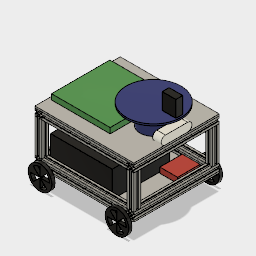
TEST AREA Body (v1~recovered) (Autodesk Fusion 360 design; units mm, degrees)
Autodesk Fusion 360 part; units mm, degrees
sketch "Sketch1" plane through (0, 0, 0) normal (0, 1, 0) x (1, 0, 0)
  line L0 (0, 0) -> (20, 0)
  line L1 (20, 0) -> (20, -20)
  line L2 (20, -20) -> (0, -20)
  line L3 (0, -20) -> (0, 0)
  line L4 (14, -14) -> (6, -14)
  line L5 (6, -14) -> (6, -6)
  line L6 (6, -6) -> (14, -6)
  line L7 (14, -6) -> (14, -14)
  line L8 (14, -14) -> (6, -6) construction
  line L9 (6, -14) -> (14, -6) construction
  circle A0 centre (10, -10) radius 2.1
  line L10 (10, 0) -> (13, 0)
  line L11 (10, 0) -> (7, 0)
  line L12 (7, 0) -> (7, -2)
  line L13 (13, 0) -> (13, -2)
  line L14 (13, -2) -> (10, -2)
  line L15 (13, -2) -> (16, -2)
  line L16 (7, -2) -> (4, -2)
  line L17 (2, -7) -> (2, -4)
  line L18 (0, -7) -> (2, -7)
  line L19 (0, -13) -> (2, -13)
  line L20 (2, -13) -> (2, -16)
  line L21 (7, -18) -> (4, -18)
  line L22 (7, -20) -> (7, -18)
  line L23 (13, -20) -> (13, -18)
  line L24 (13, -18) -> (16, -18)
  line L25 (18, -13) -> (18, -16)
  line L26 (20, -13) -> (18, -13)
  line L27 (20, -7) -> (18, -7)
  line L28 (18, -7) -> (18, -4)
  line L29 (18, -4) -> (4, -18)
  line L30 (2, -16) -> (16, -2)
  line L31 (18, -16) -> (4, -2)
  line L32 (2, -4) -> (16, -18)
  point P0 (10, -10)
  dimension "d1" = 20
  dimension "d2" = 20
  dimension "d3" = 8
  dimension "d4" = 8
  dimension "d5" = 4.2
  dimension "d6" = 3
  dimension "d7" = 3
  dimension "d8" = 2
  dimension "d9" = 2
  dimension "d11" = 360
  measures "d1" distance of L0.start L0.end
  measures "d2" distance of L0.start L2.end
  measures "d3" distance of L4.end L5.end
  measures "d4" distance of L5.end L6.end
  measures "d5" diameter of A0
  measures "d6" distance of L10.start L10.end
  measures "d7" distance of L10.start L11.end
  measures "d8" distance of L11.end L12.end
  measures "d9" distance of L10.end L13.end
extrude "Extrude1" add sketch "Sketch1" along normal blind 19 contours L0 L3 L5 L6 L12 L16 L17 L18 L31 L32 | L2 L3 L4 L5 L19 L20 L21 L22 L29 L30 | L0 L1 L6 L7 L13 L15 L27 L28 L29 L30 | L5 L6 A0 L31 L32 | L6 A0 L30 L31 | L5 A0 L30 L32 | L6 L7 A0 L29 L30 | L1 L2 L4 L7 L23 L24 L25 L26 L31 L32 | L4 L5 A0 L29 L30 | L7 A0 L29 L31 | L4 A0 L29 L32 | L4 L7 A0 L31 L32 makes body 1
sketch "Sketch2" plane through (0, 0, 0) normal (0, 1, 0) x (1, 0, 0)
  line L0 (-25, 0) -> (-197, 0)
  line L1 (-197, 0) -> (-197, -171)
  line L2 (-197, -171) -> (-25, -171)
  line L3 (-25, -171) -> (-25, 0)
  dimension "d14" = 172
  dimension "d15" = 171
  measures "d14" distance of L0.start L0.end
  measures "d15" distance of L0.start L2.end
extrude "Extrude2" add sketch "Sketch2" along normal blind 16 separate body makes body 2
sketch "Sketch3" plane through (0, 0, 0) normal (0, 1, 0) x (1, 0, 0)
  line L0 (100, 0) -> (125, 0)
  line L1 (125, 0) -> (125, -90)
  line L2 (125, -90) -> (100, -90)
  line L3 (100, -90) -> (100, 0)
  dimension "d18" = 25
  dimension "d19" = 90
  measures "d18" distance of L0.start L0.end
  measures "d19" distance of L0.start L2.end
extrude "Extrude3" add sketch "Sketch3" along normal blind 25 separate body makes body 3
fillet "Fillet1" radius 12.5 4 edges at (112.5, 25, 90) (112.5, 0, 90) (112.5, 25, 0) (112.5, 0, 0) on bodies 3
sketch "Sketch4" plane through (0, 0, 0) normal (0, 1, 0) x (1, 0, 0)
  circle A0 centre (200, 0) radius 12.5
  dimension "d23" = 25
  measures "d23" diameter of A0
extrude "Extrude4" add sketch "Sketch4" along normal blind 52 separate body makes body 4
sketch "Sketch5" plane through (0, 52, 0) normal (0, 1, 0) x (-1, 0, 0)
  circle A0 centre (-200, 0) radius 12.5
  circle A1 centre (-200, 0) radius 2
  dimension "d26" = 4
  measures "d26" diameter of A1
extrude "Extrude5" add sketch "Sketch5" along normal blind 12 contours A1 bodies 4
copy_body "CopyPasteBodies1" bodies 4 makes body 5
move_body "Move1" bodies 5 to x (1, 0, 0) y (0, 1, 0) z (0, 0, 1) at (60, 0, 0)
sketch "Sketch6" plane through (0, 0, 0) normal (0, 1, 0) x (1, 0, 0)
  line L0 (25, -100) -> (77, -100)
  line L1 (77, -100) -> (77, -166)
  line L2 (77, -166) -> (25, -166)
  line L3 (25, -166) -> (25, -100)
  dimension "d29" = 52
  dimension "d30" = 66
  measures "d29" distance of L0.start L0.end
  measures "d30" distance of L0.start L2.end
extrude "Extrude6" add sketch "Sketch6" along normal blind 16 separate body makes body 6
sketch "Sketch7" plane through (0, 0, 0) normal (0, 1, 0) x (1, 0, 0)
  line L0 (-125, 50) -> (43, 50)
  line L1 (43, 50) -> (43, 127)
  line L2 (43, 127) -> (-125, 127)
  line L3 (-125, 127) -> (-125, 50)
  dimension "d33" = 168
  dimension "d34" = 77
  measures "d33" distance of L0.start L0.end
  measures "d34" distance of L0.start L2.end
extrude "Extrude7" add sketch "Sketch7" along normal blind 181 separate body makes body 7
copy_body "CopyPasteBodies2" bodies 1 makes body 8
move_body "Move2" bodies 8 to x (1, 0, 0) y (0, 1, 0) z (0, 0, 1) at (0, 0, 275)
move_face "OffsetFaces1" offset 231 1 faces at (4, 19, 279.6667) on bodies 8
copy_body "CopyPasteBodies3" bodies 8 makes body 9
move_body "Move3" bodies 9 to x (1, 0, 0) y (0, 1, 0) z (0, 0, 1) at (0, 0, 220)
copy_body "CopyPasteBodies4" bodies 9 makes body 10
move_body "Move4" bodies 10 to x (1, 0, 0) y (0, 1, 0) z (0, 0, 1) at (0, 0, 90)
move_body "Move5" bodies 10 to x (1, 0, 0) y (0, 0, 1) z (0, -1, 0) at (0, 585, 585)
move_body "Align1" bodies 10 to x (1, 0, 0) y (0, 1, 0) z (0, 0, 1) at (0, 0, -310)
move_body "Move6" bodies 9 to x (1, 0, 0) y (0, 1, 0) z (0, 0, 1) at (0, 0, 23)
move_body "Align2" bodies 9 to x (1, 0, 0) y (0, 1, 0) z (0, 0, 1) at (0, 0, -13)
copy_body "CopyPasteBodies5" bodies 10 makes body 11
move_body "Move7" bodies 11 to x (1, 0, 0) y (0, 1, 0) z (0, 0, 1) at (0, 300, 0)
move_body "Align3" bodies 11 to x (1, 0, 0) y (0, 1, 0) z (0, 0, 1) at (0, -30, 0)
copy_body "CopyPasteBodies6" bodies 8 9 10 11 makes body 12 makes body 13 makes body 14 makes body 15
move_body "Move8" bodies 12 13 14 15 to x (1, 0, 0) y (0, 1, 0) z (0, 0, 1) at (-260, 0, 0)
copy_body "CopyPasteBodies7" bodies 1 makes body 16
move_body "Move9" bodies 16 to x (1, 0, 0) y (0, 1, 0) z (0, 0, 1) at (0, 0, 210)
move_body "Move10" bodies 16 to x (0, 1, 0) y (-1, 0, 0) z (0, 0, 1) at (0, 0, 0)
move_body "Align4" bodies 16 to x (1, 0, 0) y (0, 1, 0) z (0, 0, 1) at (0, -20, 65)
move_face "OffsetFaces2" offset 81 1 faces at (-19, -16, 279.6667) on bodies 16
move_body "Move11" bodies 11 to x (1, 0, 0) y (0, 1, 0) z (0, 0, 1) at (50, 0, 0)
move_body "Move12" bodies 11 to x (1, 0, 0) y (0, 1, 0) z (0, 0, 1) at (-50, 0, 0)
copy_body "CopyPasteBodies8" bodies 16 makes body 17
move_body "Move13" bodies 17 to x (1, 0, 0) y (0, 1, 0) z (0, 0, 1) at (0, 0, 230)
move_body "Move14" bodies 17 to x (1, 0, 0) y (0, 1, 0) z (0, 0, 1) at (0, 270, 0)
copy_body "CopyPasteBodies9" bodies 17 makes body 18
move_body "Move15" bodies 18 to x (1, 0, 0) y (0, 1, 0) z (0, 0, 1) at (0, 0, -230)
move_body "Move16" bodies 15 14 13 12 to x (1, 0, 0) y (0, 1, 0) z (0, 0, 1) at (90, 0, 0)
copy_body "CopyPasteBodies10" bodies 16 makes body 19
move_body "Move17" bodies 19 to x (1, 0, 0) y (0, 1, 0) z (0, 0, 1) at (0, 0, 230)
move_body "Move18" bodies 12 13 14 15 to x (1, 0, 0) y (0, 1, 0) z (0, 0, 1) at (-50, 0, 0)
move_body "Move19" bodies 12 13 14 15 to x (1, 0, 0) y (0, 1, 0) z (0, 0, 1) at (100, 0, 0)
sketch "Sketch8" plane through (0, 0, 0) normal (1, 0, 0) x (0, 0, -1)
  line L0 (0, 300) -> (-250, 300)
  line L1 (-250, 300) -> (-250, 590)
  line L2 (-250, 590) -> (0, 590)
  line L3 (0, 590) -> (0, 300)
  dimension "d40" = 250
  dimension "d41" = 290
  measures "d40" distance of L0.start L0.end
  measures "d41" distance of L0.start L2.end
extrude "Extrude8" add sketch "Sketch8" against normal blind 5 separate body makes body 20
copy_body "CopyPasteBodies11" bodies 20 makes body 21
move_body "Move20" bodies 21 to x (1, 0, 0) y (0, 1, 0) z (0, 0, 1) at (0, 0, 575)
move_body "Align5" bodies 20 to x (1, 0, 0) y (0, 1, 0) z (0, 0, 1) at (-120, -320, 275)
move_body "Align6" bodies 21 to x (1, 0, 0) y (0, 1, 0) z (0, 0, 1) at (25, -320, -300)
move_body "Align7" bodies 3 to x (1, 0, 0) y (0, 1, 0) z (0, 0, 1) at (-250, 270, 355)
move_body "Move21" bodies 3 to x (0, 1, 0) y (-1, 0, 0) z (0, 0, 1) at (120, 420, 0)
move_body "Align8" bodies 3 to x (1, 0, 0) y (0, 1, 0) z (0, 0, 1) at (25, -25, 0)
move_body "Move22" bodies 4 to x (1, 0, 0) y (0, 0, 1) z (0, -1, 0) at (0, -12.5, -12.5)
move_body "Move23" bodies 5 to x (1, 0, 0) y (0, 0, -1) z (0, 1, 0) at (0, 12.5, -12.5)
move_body "Align9" bodies 4 to x (1, 0, 0) y (0, 1, 0) z (0, 0, 1) at (60, 25, 0)
move_body "Move24" bodies 5 4 to x (1, 0, 0) y (0, 1, 0) z (0, 0, 1) at (-223, 0, 400)
move_body "Move25" bodies 4 to x (1, 0, 0) y (0, 1, 0) z (0, 0, 1) at (0, 0, 86)
move_body "Move26" bodies 5 to x (1, 0, 0) y (0, 1, 0) z (0, 0, 1) at (0, 0, -61)
move_body "Move27" bodies 4 5 to x (1, 0, 0) y (0, 1, 0) z (0, 0, 1) at (0, 220, 0)
sketch "Sketch9" plane through (0, 0, 537.5) normal (0, 0, 1) x (1, 0, 0)
  circle A0 centre (37, 232.5) radius 2
sketch "Sketch10" plane through (0, 0, 0) normal (0, 0, 1) x (1, 0, 0)
  circle A0 centre (139.9997, -0.5223) radius 35
  circle A1 centre (139.9997, -0.5223) radius 27.5
  line L0 (139.9997, -0.5223) -> (139.9997, -28.0223)
  line L1 (139.8029, -0.1972) -> (159.4452, -19.9678)
  line L2 (140.0001, -0.4283) -> (167.4997, -0.5223)
  line L3 (140.1984, -0.1983) -> (159.4452, 18.9231)
  line L4 (140, 0) -> (139.9997, 26.9777)
  line L5 (139.6731, -0.3268) -> (120.5543, 18.9231)
  line L6 (139.9999, -0.6233) -> (112.4997, -0.5223)
  line L7 (140.3283, -0.3284) -> (120.5543, -19.9678)
  circle A2 centre (139.9997, -0.5223) radius 2.5
  dimension "d44" = 70
  dimension "d45" = 55
  dimension "d47" = 360
  dimension "d48" = 5
  measures "d44" diameter of A0
  measures "d45" diameter of A1
  measures "d48" diameter of A2
extrude "Extrude9" add sketch "Sketch10" along normal blind 10 separate body contours A0 | A1 L1 L2 A2 | A1 L3 L4 A2 | A1 L0 L7 A2 | A1 L5 L6 A2 makes body 22
copy_body "CopyPasteBodies13" bodies 22 makes body 23
move_body "Move29" bodies 23 to x (1, 0, 0) y (0, 1, 0) z (0, 0, 1) at (60, 0, 0)
copy_body "CopyPasteBodies14" bodies 22 makes body 24
move_body "Move30" bodies 24 to x (1, 0, 0) y (0, 1, 0) z (0, 0, 1) at (130, 0, 0)
copy_body "CopyPasteBodies15" bodies 22 makes body 25
move_body "Move31" bodies 25 to x (1, 0, 0) y (0, 1, 0) z (0, 0, 1) at (200, 0, 0)
move_body "Align10" bodies 22 to x (1, 0, 0) y (0, 1, 0) z (0, 0, 1) at (-102.9997, 8.0223, 252.5)
move_body "Align11" bodies 23 to x (1, 0, 0) y (0, 1, 0) z (0, 0, 1) at (-162.9997, 8.0223, 537.5)
move_body "Align12" bodies 25 to x (1, 0, 0) y (0, 1, 0) z (0, 0, 1) at (-302.9997, 233.0223, 527.5)
move_body "Align13" bodies 24 to x (1, 0, 0) y (0, 1, 0) z (0, 0, 1) at (-232.9997, 233.0223, 262.5)
move_body "Move32" bodies 22 to x (1, 0, 0) y (0, 1, 0) z (0, 0, 1) at (0, 0, -30)
move_body "Align14" bodies 22 to x (1, 0, 0) y (0, 1, 0) z (0, 0, 1) at (0, 0, 40)
move_body "Move33" bodies 23 to x (1, 0, 0) y (0, 1, 0) z (0, 0, 1) at (0, 0, 20)
move_body "Align15" bodies 23 to x (1, 0, 0) y (0, 1, 0) z (0, 0, 1) at (0, 0, -30)
move_body "Move34" bodies 2 to x (0, 1, 0) y (-1, 0, 0) z (0, 0, 1) at (-197, 197, 0)
move_body "Align16" bodies 2 to x (1, 0, 0) y (0, 1, 0) z (0, 0, 1) at (72, 39, 314.5)
move_body "Move35" bodies 2 to x (1, 0, 0) y (0, 1, 0) z (0, 0, 1) at (0, -50, 0)
move_body "Move36" bodies 7 to x (0, 0, 1) y (0, 1, 0) z (-1, 0, 0) at (-252, 0, -2)
move_body "Align17" bodies 7 to x (1, 0, 0) y (0, 1, 0) z (0, 0, 1) at (145, 34.5, 443)
move_body "Move37" bodies 7 to x (1, 0, 0) y (0, 1, 0) z (0, 0, 1) at (0, -30, 20)
move_body "Move38" bodies 6 to x (0, 1, 0) y (-1, 0, 0) z (0, 0, 1) at (25, -25, 0)
move_body "Align18" bodies 6 to x (1, 0, 0) y (0, 1, 0) z (0, 0, 1) at (-5, 0, 0)
move_body "Align19" bodies 6 to x (1, 0, 0) y (0, 1, 0) z (0, 0, 1) at (0, 99, 267)
move_body "Move39" bodies 6 to x (1, 0, 0) y (0, 1, 0) z (0, 0, 1) at (0, 90, 60)
sketch "Sketch11" plane through (0, 0, 0) normal (1, 0, 0) x (0, 0, -1)
  circle A0 centre (0, 0) radius 40
  dimension "d51" = 80
  measures "d51" diameter of A0
extrude "Extrude10" add sketch "Sketch11" against normal blind 55 separate body makes body 26
sketch "Sketch12" plane through (-55, 0, 0) normal (-1, 0, 0) x (0, 0, 1)
  circle A0 centre (0, 0) radius 40
  circle A1 centre (0, 0) radius 80
  dimension "d54" = 160
  measures "d54" diameter of A1
extrude "Extrude11" add sketch "Sketch12" along normal blind 5 contours A0 | A1 bodies 26
move_body "Align20" bodies 26 to x (1, 0, 0) y (0, 1, 0) z (0, 0, 1) at (-125, 125, 400)
move_body "Move40" bodies 26 to x (1, 0, 0) y (0, 1, 0) z (0, 0, 1) at (0, 78, 0)
sketch "Sketch13" plane through (0, 0, 0) normal (0, 1, 0) x (1, 0, 0)
  line L0 (0, 0) -> (40, 0)
  line L1 (40, 0) -> (40, -20)
  line L2 (40, -20) -> (0, -20)
  line L3 (0, -20) -> (0, 0)
  dimension "d57" = 40
  dimension "d58" = 20
  measures "d57" distance of L0.start L0.end
  measures "d58" distance of L0.start L2.end
extrude "Extrude12" add sketch "Sketch13" along normal blind 48 separate body makes body 27
move_body "Move41" bodies 27 to x (0, 1, 0) y (-1, 0, 0) z (0, 0, 1) at (0, 0, 0)
move_body "Align21" bodies 27 to x (1, 0, 0) y (0, 1, 0) z (0, 0, 1) at (-185, 183, 390)
move_body "Move42" bodies 27 to x (1, 0, 0) y (0, 1, 0) z (0, 0, 1) at (0, 55, 0)
sketch "Sketch14" plane through (0, 0, 0) normal (0, 1, 0) x (1, 0, 0)
move_body "Move43" bodies 6 to x (1, 0, 0) y (0, 1, 0) z (0, 0, 1) at (0, 0, -125)
sketch "Sketch15" plane through (0, 0, 0) normal (0, 0, 1) x (1, 0, 0)
move_body "Move44" bodies 2 1 3 4 5 6 7 26 27 to x (0, -1, 0) y (1, 0, 0) z (0, 0, 1) at (45, 5, 0)
move_body "Move45" bodies 11 8 9 10 to x (0, -1, 0) y (1, 0, 0) z (0, 0, 1) at (45, 5, 0)
move_body "Move46" bodies 15 12 13 14 to x (0, -1, 0) y (1, 0, 0) z (0, 0, 1) at (45, 5, 0)
move_body "Move47" bodies 19 16 17 18 to x (0, -1, 0) y (1, 0, 0) z (0, 0, 1) at (45, 5, 0)
move_body "Move48" bodies 22 23 24 25 to x (0, -1, 0) y (1, 0, 0) z (0, 0, 1) at (45, 5, 0)
move_body "Move49" bodies 20 21 to x (0, -1, 0) y (1, 0, 0) z (0, 0, 1) at (45, 5, 0)
hidden bodies 1
equation "d37 = 250 mm - 19 mm"
equation "d39 = 181 mm - 100 mm"
named bodies: "Extrusion", "Jetson (green)", "Realsense (white)", "DC Motor 1 (gray)", "DC Motor 1", "DC Motor 2 (gray)", "TM4C (red)", "Battery (black)", "Extrusion (1)", "Extrusion (1) (1)", "Extrusion (1) (1) (1)", "Extrusion (1) (1) (1) (1)", "Extrusion (1) (2)", "Extrusion (1) (1) (2)", "Extrusion (1) (1) (1) (1) (1)", "Extrusion (1) (1) (1) (1) (1) (1)", "Extrusion (2)", "Extrusion (2) (1)", "Extrusion (2) (1) (1)", "Extrusion (2) (2)", "Layer", "Layer (1)", "Wheel", "Wheel (1)", "Wheel (1) (1)", "Wheel (2)", "Lidar Platform (blue)", "Lidar (black)"
